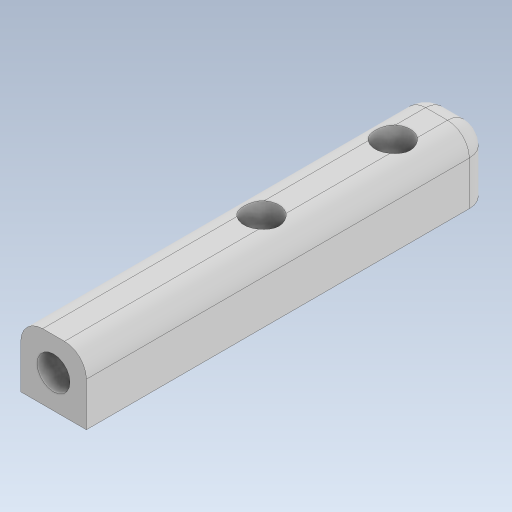
# Autodesk Inventor part: Holder Pendorong
Saved by Autodesk Inventor 2023.5 (Build 275446000, 446)
## iProperties
Created: 2025-10-17
Part Number: Holder Pendorong
Material: Generic
Document SubType Name: Modeling
Designer: Guntur
Density: 1 g/cm^3
Appearance: Default
Author: Guntur
## iProperties of the stored document Holder Pendorong_3DPrint.ipt
Created: 2025-10-18
Part Number: Holder Pendorong_3DPrint
Material: Generic
Document SubType Name: Modeling
Designer: Guntur
Density: 1 g/cm^3
Appearance: Default
Author: Guntur
Autodesk Inventor part; units mm, degrees
ref_plane "YZ Plane" through (0, 0, 0) normal (1, 0, 0) x (0, 1, 0)
ref_plane "XZ Plane" through (0, 0, 0) normal (0, 1, 0) x (-1, 0, 0)
ref_plane "XY Plane" through (0, 0, 0) normal (0, 0, 1) x (1, 0, 0)
sketch "Sketch1" plane through (0, 0, 0) normal (0, 1, 0) x (-1, 0, 0)
  circle A0 centre (0, 0) radius 1.6
  circle A1 centre (0, -12) radius 1.6
  line L0 (0, 0) -> (0, 19)
  line L1 (0, 19) -> (-3, 19)
  line L2 (-3, 19) -> (-3, -18)
  line L3 (-3, -18) -> (0, -18)
  line L4 (0, -18) -> (0, 19)
  line L5 (0, 19) -> (3, 19)
  line L6 (3, 19) -> (3, -18)
  line L7 (3, -18) -> (0, -18)
  line L8 (0, -18) -> (0, 19)
  dimension "d0" = 3.2
  dimension "d1" = 3.2
  dimension "d2" = 12
  dimension "d3" = 19
  dimension "d7" = 3
  dimension "d8" = 3
  constraints: 18 end point, 4 parallel, 2 centre point, 2 horizontal, 2 perpendicular, 1 coincident, 1 vertical
  measures "d0" diameter of A0
  measures "d1" diameter of A1
  measures "d2" distance of A1.centre point (0, 0)
  measures "d3" distance of L0.start L0.end
  measures "d7" distance of L2.end L3.end
  measures "d8" distance of L6.end L7.end
extrude "Extrusion1" add sketch "Sketch1" along normal blind 6 contours A0 L0 L5 L6 L7 L4 A1 | A0 L4 A1 L3 L2 L1 L0
sketch "Sketch2" plane through (-3, 0, 19) normal (0, 0, 1) x (1, 0, 0)
  circle A0 centre (3, 3) radius 1.5
  point P0 (3, 0)
  dimension "d9" = 3
  constraints: 1 centre point
  measures "d9" diameter of A0
extrude "Extrusion2" cut sketch "Sketch2" against normal blind 10
fillet "Fillet1" radius 2 5 edges at (3, 3, -18) (-3, 3, -18) (0, 6, -18) (3, 6, 0.5) (-3, 6, 0.5)
body "Solid1"
